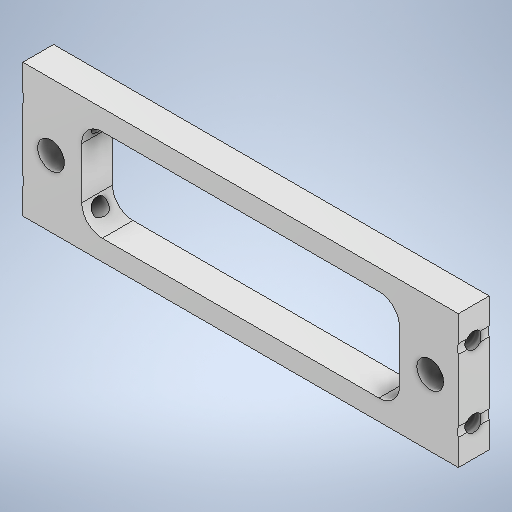
# Autodesk Inventor part: mount
Saved by Autodesk Inventor 2025.1 (Build 291241000, 241)
## iProperties
Created: 2024-09-08
Part Number: mount
Material: アルミニウム 2014-T4
Document SubType Name: Modeling
Designer: right
Density: 2.8 g/cm^3
Appearance: サテン
Mass: 2.10523 g
Surface Area: 12.4826 cm^2
Volume: 0.751867 cm^3
Author: right
Autodesk Inventor part; units mm, degrees
ref_plane "YZ Plane" through (0, 0, 0) normal (1, 0, 0) x (0, 1, 0)
ref_plane "XZ Plane" through (0, 0, 0) normal (0, 1, 0) x (-1, 0, 0)
ref_plane "XY Plane" through (0, 0, 0) normal (0, 0, 1) x (1, 0, 0)
sketch "スケッチ1" plane through (0, 0, 0) normal (0, 0, 1) x (1, 0, 0)
  circle A0 centre (-18.5, 0) radius 1.3
  circle A1 centre (18.5, 0) radius 1.3
  circle A2 centre (-18.5, 0) radius 2.75
  circle A3 centre (18.5, 0) radius 2.75
  line L0 (-21.25, 6.5) -> (21.25, 6.5)
  line L1 (21.25, 6.5) -> (21.25, -6.5)
  line L2 (21.25, -6.5) -> (-21.25, -6.5)
  line L3 (-21.25, -6.5) -> (-21.25, 6.5)
  point P0 (0, 0)
  point P1 (-21.25, 0)
  dimension "d0" = 2.6
  dimension "d1" = 2.6
  dimension "d2" = 37
  dimension "d3" = 18.5
  dimension "d6" = 13
  dimension "d45" = 42.5
  constraints: 8 end point, 4 centre point, 3 horizontal alignment, 2 coincident, 2 parallel, 2 tangent, 1 equal radius, 1 horizontal, 1 midpoint, 1 perpendicular
  measures "d0" diameter of A0
  measures "d1" diameter of A1
  measures "d2" distance of A1.centre A0.centre
  measures "d3" distance of point (0, 0) A0.centre
  measures "d6" distance of L2.end L0.start
  measures "d45" distance of L0.start L0.end
extrude "押し出し1" add sketch "スケッチ1" along normal blind 3 contours A2 | A3 | L3 L0 L1 L2
sketch "スケッチ2" plane through (0, 0, 3) normal (0, 0, 1) x (1, 0, 0)
  line L0 (-15.5, -4.5) -> (15.5, -4.5)
  line L1 (15.5, -4.5) -> (15.5, 4.5)
  line L2 (15.5, 4.5) -> (-15.5, 4.5)
  line L3 (-15.5, 4.5) -> (-15.5, -4.5)
  line L4 (-15.5, -4.5) -> (15.5, 4.5) construction
  line L5 (15.5, -4.5) -> (-15.5, 4.5) construction
  line L6 (21.25, 6.5) -> (-21.25, 6.5) projected
  circle A0 centre (-18.5, 0) radius 1.3 projected
  point P0 (0, 0)
  dimension "d9" = 2
  dimension "d10" = 3
  constraints: 12 end point, 2 midpoint, 2 parallel, 1 horizontal, 1 perpendicular
  measures "d9" distance between parallel lines of L6 L2
  measures "d10" distance from line of A0.centre L3
extrude "押し出し2" cut sketch "スケッチ2" against normal through all contours L3 L2 L1 L0
fillet "フィレット3" radius 2 4 edges at (-15.5, -4.5, 1.5) (-15.5, 4.5, 1.5) (15.5, 4.5, 1.5) (15.5, -4.5, 1.5)
sketch "スケッチ9" plane through (21.25, -6.5, 0) normal (1, 0, 0) x (0, 0, -1)
  line L0 (0, 13) -> (-3, 13) projected
  line L1 (0, 0) -> (-3, 0) projected
  line L2 (0, 6.5) -> (-3, 6.5) construction
  line L3 (-3, 4) -> (-3, 9) construction
  point P0 (-1.5, 3)
  point P1 (-1.5, 10)
  point P2 (-1.5, 13)
  point P3 (-1.5, 0)
  dimension "d46" = 3
  constraints: 3 midpoint, 2 end point, 2 vertical alignment, 1 symmetric about line
  measures "d46" distance from line of L0 point (-1.5, 10)
hole "穴1" at (21.25, -3.5, 1.5) at (21.25, 3.5, 1.5) direction (-1, 0, 0) diameter 1.567 depth 6.3 tip angle 118 thread size "M2x0.4" class "6H" standard "ISO Metric profile"
sketch "スケッチ10" plane through (-21.25, -6.5, 0) normal (-1, 0, 0) x (0, 0, 1)
  arc A0 (2.1866, 10.3775) -> (0.8134, 10.3775) centre (1.5, 10) ccw projected
  line L0 (3, 4) -> (0, 2)
  circle A1 centre (1.5, 3) radius 0.7835 projected
  point P0 (0, 6.5)
  constraints: 2 coincident, 2 end point, 1 midpoint
hole "穴2" at (-21.25, 3.5, 1.5) at (-21.25, -3.5, 1.5) direction (1, 0, 0) diameter 1.567 depth 6.3 tip angle 118 thread size "M2x0.4" class "6H" standard "ISO Metric profile"
sketch "スケッチ11" plane through (0, 0, 3) normal (0, 0, 1) x (1, 0, 0)
  circle A0 centre (-22.25, 3.5) radius 1.1
  line L0 (-21.25, 2.7165) -> (-21.25, 4.2835) construction
  line L1 (0, 0) -> (-21.25, 0) construction
  line L2 (-21.25, 6.5) -> (-21.25, -6.5) construction
  line L3 (0, 0) -> (0, 6.5) construction
  line L4 (21.25, 6.5) -> (-21.25, 6.5) construction
  circle A1 centre (22.25, 3.5) radius 1.1
  circle A2 centre (-22.25, -3.5) radius 1.1
  circle A3 centre (22.25, -3.5) radius 1.1
  point P0 (-21.25, 3.5)
  dimension "d61" = 2.2
  dimension "d62" = 1
  constraints: 4 centre point, 4 end point, 3 midpoint, 3 symmetric about line, 1 horizontal alignment, 3 other
  measures "d61" diameter of A0
  measures "d62" distance from line of L0 A0.centre
extrude "押し出し8" cut sketch "スケッチ11" against normal through all
equation "\"d1\" = d0"
equation "\"d3\" = 0.5 * d2"
